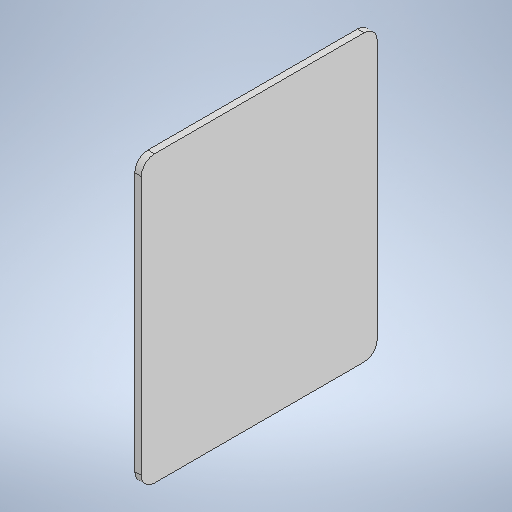
# Autodesk Inventor part: MSC 087 bottom plate gills
Saved by Autodesk Inventor 2025 (Build 290162010, 162A)
## iProperties
Created: 2024-08-30
Part Number: MSC 087 bottom plate gills
Material: Stainless Steel
Document SubType Name: Sheet Metal
Designer: pokla
Density: 8 g/cm^3
Sheet Metal Rule: AISI304 3mm Die 32
Appearance: Default
Stock Number: МОО 087 пластина опоры на дно жабры
Mass: 334.914 g
Surface Area: 293.041 cm^2
Volume: 41.8643 cm^3
Flat Pattern Width: 10.7582 cm
Flat Pattern Length: 13 cm
Flat Pattern Area: 139.857 cm^2
Sheet Metal Width: 107,582 mm
Sheet Metal Length: 130,000 mm
Sheet Metal Area: 13985,660 mm^2
Author: pokla
Autodesk Inventor part; units mm, degrees
ref_plane "YZ Plane" through (0, 0, 0) normal (1, 0, 0) x (0, 1, 0)
ref_plane "XZ Plane" through (0, 0, 0) normal (0, 1, 0) x (-1, 0, 0)
ref_plane "XY Plane" through (0, 0, 0) normal (0, 0, 1) x (1, 0, 0)
sketch "Sketch1" plane through (0, 0, 0) normal (1, 0, 0) x (0, 1, 0)
  line L0 (107.582, 130) -> (0, 130)
  line L1 (0, 130) -> (0, 0)
  line L2 (0, 0) -> (107.582, 0)
  line L3 (107.582, 0) -> (107.582, 130)
  dimension "d0" = 130
  dimension "d1" = 107.582
  measures "d0" distance of L2.end L0.start
  measures "d1" distance between parallel lines of L1 L3
extrude "Plate1" add sketch "Sketch1" along normal blind 3
fillet "Corner Round1" radius 6 4 edges at (1.5, 107.582, 130) (1.5, 107.582, 0) (1.5, 0, 130) (1.5, 0, 0)
equation "\"d2\" = Thickness"
equation "\"BendReliefWidth\" = Thickness"
equation "\"BendReliefDepth\" = 0.5 * Thickness"
equation "\"CornerReliefSize\" = 4 * Thickness"
equation "\"MinimumRemnant\" = 2 * Thickness"
equation "\"TransitionRadius\" = BendRadius"
equation "\"JacobiRadiusSize\" = BendRadius"
equation "\"GapSize\" = Thickness"
equation "\"Thickness\" = 3"
equation "\"BendRadius\" = 5"
body "Solid1"
